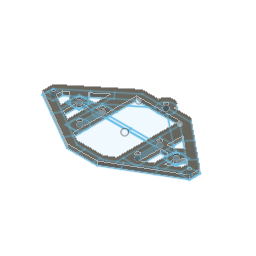
carBodyServoPlate v2 (Autodesk Fusion 360 design; units mm, degrees)
Autodesk Fusion 360 part; units mm, degrees
sketch "Sketch1" plane through (0, 0, 0) normal (0, 0, 1) x (1, 0, 0)
  line L0 (-0.0001, 25.5) -> (-0.0001, 31.5)
  circle A0 centre (-0.0001, 31.5) radius 1.65
  circle A1 centre (-0.0001, 31.5) radius 6
  line L1 (37.0364, 2.2639) -> (-37.0366, 2.2639)
  circle A2 centre (37.0364, 2.2639) radius 1.65
  circle A3 centre (-37.0366, 2.2639) radius 1.65
  line L2 (-0.0001, 31.5) -> (37.0364, 2.2639)
  line L3 (-0.0001, 31.5) -> (-37.0366, 2.2639)
  line L4 (56, 1.4) -> (56, -6.6)
  line L5 (-56, -6.6) -> (-56, 1.4)
  line L6 (-18.5, 31.9382) -> (18.5, 31.9382)
  line L7 (11.4999, -32.5) -> (-11.5001, -32.5)
  line L8 (-11.5001, -32.5) -> (-56, -6.6)
  line L9 (11.4999, -32.5) -> (56, -6.6)
  line L10 (56, -2.6) -> (52, -2.6)
  circle A4 centre (52, -2.6) radius 1.1
  line L11 (-56, -2.6) -> (-52, -2.6)
  circle A5 centre (-52, -2.6) radius 1.1
  line L12 (-22.0001, 4.7639) -> (-22.0001, 2.2639)
  line L13 (-0.0001, 2.2639) -> (-22.0001, 2.2639)
  line L14 (-22.0001, 2.2639) -> (-22.0001, 4.7639)
  line L15 (-22.0001, 4.7639) -> (-0.0001, 4.7639)
  line L16 (-0.0001, 4.7639) -> (-0.0001, 2.2639)
  line L17 (-0.0001, 4.7639) -> (21.9999, 4.7639)
  line L18 (21.9999, 4.7639) -> (21.9999, 2.2639)
  line L19 (21.9999, 2.2639) -> (-0.0001, 2.2639)
  line L20 (-0.0001, 2.2639) -> (-0.0001, 4.7639)
  circle A6 centre (-22.0001, 4.7639) radius 1.65
  circle A7 centre (21.9999, 4.7639) radius 1.65
  line L21 (21.9999, 4.7639) -> (21.9999, -12.2361)
  line L22 (-22.0001, 4.7639) -> (-22.0001, -12.2361)
  circle A8 centre (21.9999, -12.2361) radius 1.65
  circle A9 centre (-22.0001, -12.2361) radius 1.65
  circle A10 centre (-22.0001, -12.2361) radius 5.5
  circle A11 centre (-22.0001, 4.7639) radius 5.5
  line L23 (-27.5001, -17.7361) -> (-16.5001, -17.7361)
  line L24 (-16.5001, -17.7361) -> (-16.5001, 10.2639)
  line L25 (-16.5001, 10.2639) -> (-27.5001, 10.2639)
  line L26 (-27.5001, 10.2639) -> (-27.5001, -17.7361)
  line L27 (27.4999, -17.7361) -> (27.4999, 10.2639)
  line L28 (27.4999, 10.2639) -> (16.4999, 10.2639)
  line L29 (16.4999, 10.2639) -> (16.4999, -17.7361)
  line L30 (16.4999, -17.7361) -> (27.4999, -17.7361)
  line L31 (56, -6.6) -> (48, -6.6)
  line L32 (48, -6.6) -> (48, 1.4)
  line L33 (48, 1.4) -> (56, 1.4)
  line L34 (56, 1.4) -> (56, -6.6)
  line L35 (-56, -6.6) -> (-48, -6.6)
  line L36 (-48, -6.6) -> (-48, 1.4)
  line L37 (-48, 1.4) -> (-56, 1.4)
  line L38 (-56, 1.4) -> (-56, -6.6)
  line L39 (-20.5229, -27.2485) -> (-17.5048, -22.0629)
  line L40 (-40.4384, -15.6572) -> (-37.4202, -10.4716)
  line L41 (-17.5048, -22.0629) -> (-37.4202, -10.4716)
  line L42 (-37.4202, -10.4716) -> (-48, -4.3139)
  line L43 (-17.5048, -22.0629) -> (-11.5001, -25.5578)
  line L44 (22.8887, -25.8715) -> (19.8706, -20.6859)
  line L45 (39.4309, -16.2436) -> (36.4127, -11.058)
  line L46 (36.4127, -11.058) -> (19.8706, -20.6859)
  line L47 (36.4127, -11.058) -> (48, -4.3139)
  line L48 (19.8706, -20.6859) -> (11.4999, -25.5578)
  line L49 (56, 1.4) -> (18.5, 31.9382)
  line L50 (45.76, 9.7389) -> (41.9713, 5.0865)
  line L51 (31.8969, 21.0284) -> (28.1081, 16.376)
  line L52 (41.9713, 5.0865) -> (28.1081, 16.376)
  line L53 (28.1081, 16.376) -> (15.6762, 26.5)
  line L54 (41.9713, 5.0865) -> (48, 0.177)
  circle A12 centre (37.0364, 2.2639) radius 5
  line L55 (32.0364, -2.7361) -> (42.0364, -2.7361)
  line L56 (42.0364, -2.7361) -> (42.0364, 7.2639)
  line L57 (42.0364, 7.2639) -> (32.0364, 7.2639)
  line L58 (32.0364, 7.2639) -> (32.0364, -2.7361)
  line L59 (42.0364, -2.7361) -> (37.0364, 2.2639)
  line L60 (32.0364, 7.2639) -> (37.0364, 2.2639)
  line L61 (40.572, -1.2717) -> (44.2431, 3.2364)
  line L62 (33.5009, 5.7994) -> (36.9098, 9.2083)
  line L63 (-56, 1.4) -> (-18.5, 31.9382)
  line L64 (-30.0227, 22.5547) -> (-26.234, 17.9022)
  line L65 (-40.3156, 14.1727) -> (-36.5979, 9.4632)
  line L66 (-26.234, 17.9022) -> (-36.5979, 9.4632)
  line L67 (-36.5979, 9.4632) -> (-48, 0.4625)
  line L68 (-26.234, 17.9022) -> (-15.6762, 26.5)
  line L69 (7.8699, -32.5) -> (7.8699, -26.5)
  line L70 (-4.112, -32.5) -> (-4.112, -26.5)
  line L71 (7.8699, -26.5) -> (-4.112, -26.5)
  line L72 (11.4999, -25.5578) -> (9.881, -26.5)
  line L73 (9.881, -26.5) -> (7.8699, -26.5)
  line L74 (-4.112, -26.5) -> (-9.8811, -26.5)
  line L75 (-9.8811, -26.5) -> (-11.5001, -25.5578)
  line L76 (16.4999, -17.7361) -> (16.4999, -22.6477)
  line L77 (-16.5001, -17.7361) -> (-16.5001, -22.6477)
  line L78 (27.4999, 10.2639) -> (27.4999, 16.8713)
  line L79 (-27.5001, 10.2639) -> (-27.5001, 16.8713)
  line L80 (-0.0001, 25.5) -> (16.9042, 25.5)
  line L81 (16.4999, 10.2639) -> (16.4999, 25.5)
  line L82 (-0.0001, 25.5) -> (-16.9042, 25.5)
  line L83 (-16.5001, 10.2639) -> (-16.5001, 25.5)
  line L84 (-42.0366, 7.2639) -> (-37.0366, 7.2639)
  line L85 (-37.0366, 7.2639) -> (-37.0366, 2.2639)
  line L86 (-32.0366, -2.7361) -> (-42.0366, -2.7361)
  line L87 (-42.0366, -2.7361) -> (-42.0366, 7.2639)
  line L88 (-42.0366, 7.2639) -> (-32.0366, 7.2639)
  line L89 (-32.0366, 7.2639) -> (-32.0366, -2.7361)
  line L90 (-32.0366, 7.2639) -> (-42.0366, -2.7361)
  circle A13 centre (-37.0366, 2.2639) radius 5
  line L91 (-33.501, 5.7994) -> (-36.9147, 9.2131)
  line L92 (-40.5721, -1.2717) -> (-44.8181, 2.9743)
  line L93 (37.0364, -2.7361) -> (34.5364, -2.7361)
  line L94 (37.0364, -2.7361) -> (39.5364, -2.7361)
  line L95 (39.5364, -2.7361) -> (39.5364, -9.2399)
  line L96 (39.5364, -2.7361) -> (39.5364, -2.0663)
  line L97 (34.5364, -2.7361) -> (34.5364, -2.0663)
  line L98 (34.5364, -2.7361) -> (34.5364, -12.15)
  line L99 (32.0364, 2.2639) -> (32.0364, 4.7639)
  line L100 (32.0364, 4.7639) -> (27.4999, 4.7639)
  line L101 (32.0364, 2.2639) -> (32.0364, -0.2361)
  line L102 (32.0364, -0.2361) -> (27.4999, -0.2361)
  line L103 (32.0364, -0.2361) -> (32.7063, -0.2361)
  line L104 (32.0364, 4.7639) -> (32.7063, 4.7639)
  line L105 (-32.0366, -0.2361) -> (-27.5001, -0.2361)
  line L106 (-32.0366, 4.7639) -> (-27.5001, 4.7639)
  line L107 (-32.0366, 4.7639) -> (-32.7064, 4.7639)
  line L108 (-32.0366, -0.2361) -> (-32.7064, -0.2361)
  line L109 (-37.0366, -2.7361) -> (-39.5366, -2.7361)
  line L110 (-37.0366, -2.7361) -> (-34.5366, -2.7361)
  line L111 (-34.5366, -2.7361) -> (-34.5366, -12.15)
  line L112 (-39.5366, -2.7361) -> (-39.5366, -9.2398)
  line L113 (23.6499, -12.2361) -> (20.3499, -12.2361)
  line L114 (20.3499, -12.2361) -> (20.3499, 4.7639)
  line L115 (20.3499, 4.7639) -> (23.6499, 4.7639)
  line L116 (23.6499, 4.7639) -> (23.6499, -12.2361)
  line L117 (-20.3501, -12.2361) -> (-23.6501, -12.2361)
  line L118 (-23.6501, -12.2361) -> (-23.6501, 4.7639)
  line L119 (-23.6501, 4.7639) -> (-20.3501, 4.7639)
  line L120 (-20.3501, 4.7639) -> (-20.3501, -12.2361)
  line L121 (-34.5366, -2.7361) -> (-34.5366, -2.0663)
  line L122 (-39.5366, -2.7361) -> (-39.5366, -2.0663)
  dimension "d3" = 6
  dimension "d4" = 3.3
  dimension "d5" = 12
  dimension "d20" = 3.3
  dimension "d21" = 3.3
  dimension "d24" = 112
  dimension "d25" = 8
  dimension "d26" = 37
  dimension "d30" = 2.2
  dimension "d31" = 4
  dimension "d32" = 4
  dimension "d33" = 2.2
  dimension "d36" = 22
  dimension "d37" = 2.5
  dimension "d38" = 22
  dimension "d39" = 2.5
  dimension "d41" = 3.3
  dimension "d42" = 3.3
  dimension "d58" = 17
  dimension "d59" = 17
  dimension "d60" = 3.3
  dimension "d61" = 3.3
  dimension "d62" = 11
  dimension "d63" = 11
  dimension "d64" = 8
  dimension "d65" = 8
  dimension "d66" = 6
  dimension "d67" = 6
  dimension "d68" = 6
  dimension "d69" = 6
  dimension "d70" = 6
  dimension "d71" = 6
  dimension "d72" = 10
  dimension "d73" = 6
  dimension "d74" = 6
  dimension "d75" = 6
  dimension "d76" = 6
  dimension "d79" = 5
  dimension "d82" = 10
  dimension "d83" = 2.5
  dimension "d84" = 2.5
  dimension "d85" = 2.5
  dimension "d86" = 2.5
  dimension "d87" = 2.5
  dimension "d88" = 2.5
  constraint coincident L0.end A0.centre
  constraint coincident L1.start A2.centre
  constraint coincident L1.end A3.centre
  constraint vertical L4
  constraint vertical L5
  constraint horizontal L6
  constraint horizontal L7
  constraint midpoint L4 L10.start
  constraint perpendicular L4 L10
  constraint coincident L10.end A4.centre
  constraint midpoint L5 L11.start
  constraint perpendicular L5 L11
  constraint coincident L11.end A5.centre
  constraint coincident L1 L12.end
  constraint perpendicular L1 L12
  constraint horizontal L13
  constraint vertical L14
  constraint horizontal L15
  constraint vertical L16
  constraint midpoint L1 L13.start
  constraint horizontal L17
  constraint vertical L18
  constraint horizontal L19
  constraint vertical L20
  constraint coincident L17.end L18.start
  constraint perpendicular L1 L21
  constraint coincident L12.start L14.end
  constraint perpendicular L13 L22
  constraint coincident L21.end A8.centre
  constraint coincident L22.end A9.centre
  constraint concentric A9 A10
  constraint concentric A6 A11
  constraint horizontal L23
  constraint vertical L24
  constraint horizontal L25
  constraint vertical L26
  constraint horizontal L30
  constraint vertical L27
  constraint horizontal L28
  constraint vertical L29
  constraint horizontal L31
  constraint vertical L32
  constraint horizontal L33
  constraint vertical L34
  constraint horizontal L35
  constraint vertical L36
  constraint horizontal L37
  constraint vertical L38
  constraint coincident L8 L39.start
  constraint perpendicular L8 L39
  constraint coincident L8 L40.start
  constraint perpendicular L8 L40
  constraint perpendicular L40 L41
  constraint coincident L36 L42.end
  constraint perpendicular L40 L42
  constraint perpendicular L39 L43
  constraint coincident L9 L44.start
  constraint perpendicular L9 L44
  constraint coincident L9 L45.start
  constraint perpendicular L9 L45
  constraint perpendicular L44 L46
  constraint coincident L32 L47.end
  constraint perpendicular L45 L47
  constraint perpendicular L44 L48
  constraint coincident L49 L50.start
  constraint perpendicular L49 L50
  constraint coincident L49 L51.start
  constraint perpendicular L49 L51
  constraint perpendicular L51 L52
  constraint perpendicular L51 L53
  constraint coincident L32 L54.end
  constraint perpendicular L50 L54
  constraint concentric A2 A12
  constraint horizontal L55
  constraint vertical L56
  constraint horizontal L57
  constraint vertical L58
  constraint parallel L59 L60
  constraint coincident L59 L61.start
  constraint coincident A12 L61.start
  constraint coincident L54 L61.end
  constraint perpendicular L54 L61
  constraint coincident L60 L62.start
  constraint coincident A12 L62.start
  constraint coincident L52 L62.end
  constraint tangent A12 L62
  constraint coincident L63 L64.start
  constraint perpendicular L63 L64
  constraint coincident L63 L65.start
  constraint perpendicular L3 L65
  constraint coincident L36 L67.end
  constraint perpendicular L65 L67
  constraint perpendicular L64 L68
  constraint coincident L7 L69.start
  constraint perpendicular L7 L69
  constraint coincident L7 L70.start
  constraint perpendicular L7 L70
  constraint perpendicular L70 L71
  constraint parallel L9 L72
  constraint perpendicular L69 L73
  constraint perpendicular L70 L74
  constraint parallel L43 L75
  constraint coincident L48 L76.end
  constraint perpendicular L30 L76
  constraint coincident L43 L77.end
  constraint perpendicular L23 L77
  constraint coincident L53 L78.end
  constraint perpendicular L28 L78
  constraint coincident L66 L79.end
  constraint perpendicular L25 L79
  constraint coincident L53 L80.end
  constraint tangent A1 L80
  constraint coincident L80 L81.end
  constraint perpendicular L80 L81
  constraint coincident L68 L82.end
  constraint tangent A1 L82
  constraint coincident L82 L83.end
  constraint perpendicular L82 L83
  constraint horizontal L84
  constraint vertical L85
  constraint horizontal L86
  constraint vertical L87
  constraint horizontal L88
  constraint vertical L89
  constraint concentric A3 A13
  constraint coincident A13 L91.start
  constraint coincident L90 L91.start
  constraint coincident L67 L91.end
  constraint tangent A13 L91
  constraint perpendicular L90 L91
  constraint coincident A13 L92.start
  constraint coincident L90 L92.start
  constraint coincident L67 L92.end
  constraint tangent A13 L92
  constraint midpoint L55 L93.start
  constraint parallel L55 L93
  constraint parallel L55 L94
  constraint coincident L47 L95.end
  constraint perpendicular L94 L95
  constraint coincident A12 L96.end
  constraint perpendicular L94 L96
  constraint coincident A12 L97.end
  constraint perpendicular L93 L97
  constraint coincident L46 L98.end
  constraint perpendicular L93 L98
  constraint midpoint L58 L99.start
  constraint perpendicular L1 L99
  constraint coincident L27 L100.end
  constraint perpendicular L27 L100
  constraint perpendicular L100 L101
  constraint coincident L27 L102.end
  constraint perpendicular L27 L102
  constraint coincident A12 L103.end
  constraint perpendicular L58 L103
  constraint coincident A12 L104.end
  constraint perpendicular L99 L104
  constraint coincident L89 L105.start
  constraint coincident L26 L105.end
  constraint perpendicular L26 L105
  constraint coincident L89 L106.start
  constraint coincident L26 L106.end
  constraint coincident A11 L106.end
  constraint perpendicular L26 L106
  constraint coincident A13 L107.end
  constraint perpendicular L89 L107
  constraint coincident A13 L108.end
  constraint perpendicular L89 L108
  constraint midpoint L86 L109.start
  constraint perpendicular L26 L109
  constraint parallel L86 L110
  constraint coincident L41 L111.end
  constraint perpendicular L110 L111
  constraint coincident L42 L112.end
  constraint perpendicular L109 L112
  constraint horizontal L113
  constraint vertical L114
  constraint horizontal L115
  constraint vertical L116
  constraint coincident A7 L114.end
  constraint coincident L17 L114.end
  constraint coincident A8 L113.start
  constraint horizontal L117
  constraint vertical L118
  constraint horizontal L119
  constraint vertical L120
  constraint coincident A6 L118.end
  constraint coincident A9 L117.start
  constraint coincident A13 L121.end
  constraint perpendicular L86 L121
  constraint coincident A13 L122.end
  constraint perpendicular L86 L122
  measures "d3" distance of L0.start L0.end
  measures "d4" diameter of A0
  measures "d5" diameter of A1
  measures "d20" diameter of A2
  measures "d21" diameter of A3
  measures "d24" distance of L5.end L4.start
  measures "d25" distance of L5.end L5.start
  measures "d26" distance of L6.start L6.end
  measures "d30" diameter of A4
  measures "d31" distance of L10.start L10.end
  measures "d32" distance of L11.start L11.end
  measures "d33" diameter of A5
  measures "d36" distance of L12.start L15.end
  measures "d37" distance of L13.start L15.end
  measures "d38" distance of L15.end L17.end
  measures "d39" distance of L15.end L13.start
  measures "d41" diameter of A6
  measures "d42" diameter of A7
  measures "d58" distance of L17.end L21.end
  measures "d59" distance of L12.start L22.end
  measures "d60" diameter of A8
  measures "d61" diameter of A9
  measures "d62" diameter of A10
  measures "d63" diameter of A11
  measures "d64" distance of L4.end L31.end
  measures "d65" distance of L5.start L35.end
  measures "d66" distance of L39.start L39.end
  measures "d67" distance of L40.start L40.end
  measures "d68" distance of L44.start L44.end
  measures "d69" distance of L45.start L45.end
  measures "d70" distance of L50.start L50.end
  measures "d71" distance of L51.start L51.end
  measures "d72" diameter of A12
  measures "d73" distance of L64.start L64.end
  measures "d74" distance of L65.start L65.end
  measures "d75" distance of L69.start L69.end
  measures "d76" distance of L70.start L70.end
  measures "d79" distance of L1.end L84.end
  measures "d82" diameter of A13
  measures "d83" distance of L93.start L93.end
  measures "d84" distance of L93.start L94.end
  measures "d85" distance of L99.start L99.end
  measures "d86" distance of L99.start L101.end
  measures "d87" distance of L109.start L109.end
  measures "d88" distance of L109.start L110.end
sketch "Sketch1 (2)" plane through (0, 0, 0) normal (0, 0, 1) x (1, 0, 0) in component "carBodyServoPlate"
  line L0 (11.4999, -32.5) -> (-11.5001, -32.5)
  line L1 (-32.0366, -0.2361) -> (-27.5001, -0.2361)
  line L2 (-26.234, 17.9022) -> (-15.6762, 26.5)
  line L3 (-37.0366, 7.2639) -> (-37.0366, 2.2639)
  line L4 (-48, 1.4) -> (-56, 1.4)
  line L5 (-22.0001, 2.2639) -> (-22.0001, 4.7639)
  line L6 (-40.3156, 14.1727) -> (-36.5979, 9.4632)
  circle A0 centre (-22.0001, 4.7639) radius 1.65
  line L7 (-0.0001, 25.5) -> (-16.9042, 25.5)
  line L8 (-32.0366, 4.7639) -> (-32.7064, 4.7639)
  line L9 (-56, 1.4) -> (-18.5, 31.9382)
  line L10 (-0.0001, 4.7639) -> (21.9999, 4.7639)
  circle A1 centre (-37.0366, 2.2639) radius 1.65
  line L11 (-32.0366, 4.7639) -> (-27.5001, 4.7639)
  line L12 (-42.0366, 7.2639) -> (-32.0366, 7.2639)
  line L13 (-36.5979, 9.4632) -> (-48, 0.4625)
  line L14 (-32.0366, -0.2361) -> (-32.7064, -0.2361)
  line L15 (27.4999, 10.2639) -> (27.4999, 16.8713)
  line L16 (37.0364, -2.7361) -> (34.5364, -2.7361)
  line L17 (39.4309, -16.2436) -> (36.4127, -11.058)
  line L18 (16.4999, -17.7361) -> (16.4999, -22.6477)
  line L19 (32.0364, 2.2639) -> (32.0364, 4.7639)
  line L20 (-34.5366, -2.7361) -> (-34.5366, -2.0663)
  line L21 (32.0364, 2.2639) -> (32.0364, -0.2361)
  line L22 (28.1081, 16.376) -> (15.6762, 26.5)
  circle A2 centre (-22.0001, -12.2361) radius 5.5
  line L23 (-40.4384, -15.6572) -> (-37.4202, -10.4716)
  line L24 (32.0364, -2.7361) -> (42.0364, -2.7361)
  line L25 (45.76, 9.7389) -> (41.9713, 5.0865)
  line L26 (31.8969, 21.0284) -> (28.1081, 16.376)
  line L27 (-34.5366, -2.7361) -> (-34.5366, -12.15)
  line L28 (42.0364, 7.2639) -> (32.0364, 7.2639)
  line L29 (-27.5001, -17.7361) -> (-16.5001, -17.7361)
  line L30 (-4.112, -26.5) -> (-9.8811, -26.5)
  line L31 (27.4999, 10.2639) -> (16.4999, 10.2639)
  line L32 (-20.5229, -27.2485) -> (-17.5048, -22.0629)
  line L33 (-20.3501, -12.2361) -> (-23.6501, -12.2361)
  line L34 (32.0364, 4.7639) -> (27.4999, 4.7639)
  line L35 (39.5364, -2.7361) -> (39.5364, -9.2399)
  circle A3 centre (-52, -2.6) radius 1.1
  circle A4 centre (-22.0001, -12.2361) radius 1.65
  line L36 (32.0364, -0.2361) -> (32.7063, -0.2361)
  line L37 (32.0364, 7.2639) -> (37.0364, 2.2639)
  line L38 (39.5364, -2.7361) -> (39.5364, -2.0663)
  line L39 (7.8699, -32.5) -> (7.8699, -26.5)
  line L40 (-16.5001, -17.7361) -> (-16.5001, -22.6477)
  line L41 (11.4999, -25.5578) -> (9.881, -26.5)
  line L42 (36.4127, -11.058) -> (48, -4.3139)
  line L43 (36.4127, -11.058) -> (19.8706, -20.6859)
  circle A5 centre (21.9999, 4.7639) radius 1.65
  line L44 (-56, -2.6) -> (-52, -2.6)
  circle A6 centre (52, -2.6) radius 1.1
  line L45 (-4.112, -32.5) -> (-4.112, -26.5)
  line L46 (32.0364, 4.7639) -> (32.7063, 4.7639)
  circle A7 centre (37.0364, 2.2639) radius 1.65
  line L47 (34.5364, -2.7361) -> (34.5364, -12.15)
  line L48 (20.3499, 4.7639) -> (23.6499, 4.7639)
  line L49 (-39.5366, -2.7361) -> (-39.5366, -9.2398)
  line L50 (33.5009, 5.7994) -> (36.9098, 9.2083)
  line L51 (23.6499, -12.2361) -> (20.3499, -12.2361)
  line L52 (41.9713, 5.0865) -> (28.1081, 16.376)
  line L53 (-32.0366, 7.2639) -> (-42.0366, -2.7361)
  line L54 (-37.0366, -2.7361) -> (-39.5366, -2.7361)
  line L55 (41.9713, 5.0865) -> (48, 0.177)
  line L56 (-11.5001, -32.5) -> (-56, -6.6)
  line L57 (22.8887, -25.8715) -> (19.8706, -20.6859)
  line L58 (-20.3501, 4.7639) -> (-20.3501, -12.2361)
  line L59 (-23.6501, -12.2361) -> (-23.6501, 4.7639)
  line L60 (-9.8811, -26.5) -> (-11.5001, -25.5578)
  line L61 (-22.0001, 4.7639) -> (-22.0001, -12.2361)
  line L62 (21.9999, 4.7639) -> (21.9999, -12.2361)
  line L63 (-56, -6.6) -> (-56, 1.4)
  line L64 (20.3499, -12.2361) -> (20.3499, 4.7639)
  line L65 (56, 1.4) -> (56, -6.6)
  line L66 (-40.5721, -1.2717) -> (-44.8181, 2.9743)
  line L67 (42.0364, -2.7361) -> (42.0364, 7.2639)
  line L68 (42.0364, -2.7361) -> (37.0364, 2.2639)
  line L69 (-56, 1.4) -> (-56, -6.6)
  line L70 (-32.0366, -2.7361) -> (-42.0366, -2.7361)
  line L71 (-39.5366, -2.7361) -> (-39.5366, -2.0663)
  line L72 (56, 1.4) -> (56, -6.6)
  line L73 (16.4999, -17.7361) -> (27.4999, -17.7361)
  line L74 (-17.5048, -22.0629) -> (-11.5001, -25.5578)
  circle A8 centre (-37.0366, 2.2639) radius 5
  line L75 (56, 1.4) -> (18.5, 31.9382)
  line L76 (-27.5001, 10.2639) -> (-27.5001, -17.7361)
  line L77 (-56, -6.6) -> (-48, -6.6)
  line L78 (-0.0001, 4.7639) -> (-0.0001, 2.2639)
  line L79 (16.4999, 10.2639) -> (16.4999, 25.5)
  line L80 (27.4999, -17.7361) -> (27.4999, 10.2639)
  line L81 (32.0364, 7.2639) -> (32.0364, -2.7361)
  line L82 (-37.4202, -10.4716) -> (-48, -4.3139)
  line L83 (-37.0366, -2.7361) -> (-34.5366, -2.7361)
  line L84 (21.9999, 4.7639) -> (21.9999, 2.2639)
  line L85 (56, -6.6) -> (48, -6.6)
  line L86 (-16.5001, -17.7361) -> (-16.5001, 10.2639)
  line L87 (48, -6.6) -> (48, 1.4)
  line L88 (-17.5048, -22.0629) -> (-37.4202, -10.4716)
  line L89 (-27.5001, 10.2639) -> (-27.5001, 16.8713)
  line L90 (21.9999, 2.2639) -> (-0.0001, 2.2639)
  line L91 (-22.0001, 4.7639) -> (-22.0001, 2.2639)
  line L92 (-23.6501, 4.7639) -> (-20.3501, 4.7639)
  line L93 (-0.0001, 25.5) -> (16.9042, 25.5)
  line L94 (-16.5001, 10.2639) -> (-16.5001, 25.5)
  line L95 (-18.5, 31.9382) -> (18.5, 31.9382)
  line L96 (19.8706, -20.6859) -> (11.4999, -25.5578)
  line L97 (48, 1.4) -> (56, 1.4)
  line L98 (37.0364, -2.7361) -> (39.5364, -2.7361)
  line L99 (11.4999, -32.5) -> (56, -6.6)
  line L100 (40.572, -1.2717) -> (44.2431, 3.2364)
  circle A9 centre (21.9999, -12.2361) radius 1.65
  line L101 (32.0364, -0.2361) -> (27.4999, -0.2361)
  line L102 (34.5364, -2.7361) -> (34.5364, -2.0663)
  line L103 (9.881, -26.5) -> (7.8699, -26.5)
  line L104 (56, -2.6) -> (52, -2.6)
  line L105 (-0.0001, 2.2639) -> (-0.0001, 4.7639)
  line L106 (-26.234, 17.9022) -> (-36.5979, 9.4632)
  line L107 (-0.0001, 25.5) -> (-0.0001, 31.5)
  circle A10 centre (-0.0001, 31.5) radius 1.65
  line L108 (-33.501, 5.7994) -> (-36.9147, 9.2131)
  line L109 (7.8699, -26.5) -> (-4.112, -26.5)
  line L110 (-30.0227, 22.5547) -> (-26.234, 17.9022)
  line L111 (-32.0366, 7.2639) -> (-32.0366, -2.7361)
  line L112 (-22.0001, 4.7639) -> (-0.0001, 4.7639)
  line L113 (-16.5001, 10.2639) -> (-27.5001, 10.2639)
  line L114 (-42.0366, 7.2639) -> (-37.0366, 7.2639)
  circle A11 centre (-0.0001, 31.5) radius 6
  line L115 (-48, -6.6) -> (-48, 1.4)
  line L116 (37.0364, 2.2639) -> (-37.0366, 2.2639)
  line L117 (-42.0366, -2.7361) -> (-42.0366, 7.2639)
  circle A12 centre (-22.0001, 4.7639) radius 5.5
  line L118 (-0.0001, 31.5) -> (-37.0366, 2.2639)
  line L119 (-0.0001, 31.5) -> (37.0364, 2.2639)
  line L120 (23.6499, 4.7639) -> (23.6499, -12.2361)
  line L121 (-0.0001, 2.2639) -> (-22.0001, 2.2639)
  line L122 (16.4999, 10.2639) -> (16.4999, -17.7361)
  circle A13 centre (37.0364, 2.2639) radius 5
  dimension "d93" = 6
  dimension "d94" = 3.3
  dimension "d95" = 12
  dimension "d96" = 3.3
  dimension "d97" = 3.3
  dimension "d98" = 112
  dimension "d99" = 8
  dimension "d100" = 37
  dimension "d101" = 2.2
  dimension "d102" = 4
  dimension "d103" = 4
  dimension "d104" = 2.2
  dimension "d105" = 22
  dimension "d106" = 2.5
  dimension "d107" = 22
  dimension "d108" = 2.5
  dimension "d109" = 3.3
  dimension "d110" = 3.3
  dimension "d111" = 17
  dimension "d112" = 17
  dimension "d113" = 3.3
  dimension "d114" = 3.3
  dimension "d115" = 11
  dimension "d116" = 11
  dimension "d117" = 8
  dimension "d118" = 8
  dimension "d119" = 6
  dimension "d120" = 6
  dimension "d121" = 6
  dimension "d122" = 6
  dimension "d123" = 6
  dimension "d124" = 6
  dimension "d125" = 10
  dimension "d126" = 6
  dimension "d127" = 6
  dimension "d128" = 6
  dimension "d129" = 6
  dimension "d130" = 5
  dimension "d131" = 10
  dimension "d132" = 2.5
  dimension "d133" = 2.5
  dimension "d134" = 2.5
  dimension "d135" = 2.5
  dimension "d136" = 2.5
  dimension "d137" = 2.5
  constraint coincident L107.end A10.centre
  constraint coincident L37.end A7.centre
  constraint coincident L3.end A1.centre
  constraint vertical L65
  constraint vertical L63
  constraint horizontal L95
  constraint horizontal L0
  constraint midpoint L104.start L65
  constraint perpendicular L65 L104
  constraint coincident A6.centre L104.end
  constraint midpoint L44.start L63
  constraint perpendicular L44 L63
  constraint coincident A3.centre L44.end
  constraint coincident L5.start L116
  constraint perpendicular L91 L116
  constraint horizontal L121
  constraint vertical L5
  constraint horizontal L112
  constraint vertical L78
  constraint midpoint L78.end L116
  constraint horizontal L10
  constraint vertical L84
  constraint horizontal L90
  constraint vertical L105
  constraint coincident L10.end A5.centre
  constraint perpendicular L62 L116
  constraint coincident L5.end A0.centre
  constraint perpendicular L61 L121
  constraint coincident L62.end A9.centre
  constraint coincident A2.centre A4.centre
  constraint concentric A2 A4
  constraint concentric A0 A12
  constraint horizontal L29
  constraint vertical L86
  constraint horizontal L113
  constraint vertical L76
  constraint horizontal L73
  constraint vertical L80
  constraint horizontal L31
  constraint vertical L122
  constraint horizontal L85
  constraint vertical L87
  constraint horizontal L97
  constraint vertical L72
  constraint horizontal L77
  constraint vertical L115
  constraint horizontal L4
  constraint vertical L69
  constraint coincident L32.start L56
  constraint perpendicular L32 L56
  constraint coincident L23.start L56
  constraint perpendicular L23 L56
  constraint perpendicular L23 L88
  constraint coincident L82.end L115
  constraint perpendicular L23 L82
  constraint perpendicular L32 L74
  constraint coincident L57.start L99
  constraint perpendicular L57 L99
  constraint coincident L17.start L99
  constraint perpendicular L17 L99
  constraint perpendicular L43 L57
  constraint coincident L42.end L87
  constraint perpendicular L17 L42
  constraint perpendicular L57 L96
  constraint coincident L25.start L75
  constraint perpendicular L25 L75
  constraint coincident L26.start L75
  constraint perpendicular L26 L75
  constraint perpendicular L26 L52
  constraint perpendicular L22 L26
  constraint coincident L55.end L87
  constraint perpendicular L25 L55
  constraint concentric A7 A13
  constraint horizontal L24
  constraint vertical L67
  constraint horizontal L28
  constraint vertical L81
  constraint parallel L37 L68
  constraint coincident L100.start L68
  constraint coincident L100.start A13
  constraint coincident L100.end L55
  constraint perpendicular L55 L100
  constraint coincident L50.start L37
  constraint coincident L50.start A13
  constraint coincident L50.end L52
  constraint tangent L50 A13
  constraint coincident L110.start L9
  constraint perpendicular L9 L110
  constraint coincident L6.start L9
  constraint perpendicular L6 L118
  constraint coincident L13.end L115
  constraint perpendicular L6 L13
  constraint perpendicular L2 L110
  constraint coincident L39.start L0
  constraint perpendicular L0 L39
  constraint coincident L45.start L0
  constraint perpendicular L0 L45
  constraint perpendicular L45 L109
  constraint parallel L41 L99
  constraint perpendicular L39 L103
  constraint perpendicular L30 L45
  constraint parallel L60 L74
  constraint coincident L18.end L96
  constraint perpendicular L18 L73
  constraint coincident L40.end L74
  constraint perpendicular L29 L40
  constraint coincident L15.end L22
  constraint perpendicular L15 L31
  constraint coincident L89.end L106
  constraint perpendicular L89 L113
  constraint coincident L93.end L22
  constraint tangent L93 A11
  constraint coincident L79.end L93
  constraint perpendicular L79 L93
  constraint coincident L7.end L2
  constraint tangent L7 A11
  constraint coincident L94.end L7
  constraint perpendicular L7 L94
  constraint horizontal L114
  constraint vertical L3
  constraint horizontal L70
  constraint vertical L117
  constraint horizontal L12
  constraint vertical L111
  constraint concentric A1 A8
  constraint coincident L108.start A8
  constraint coincident L108.start L53
  constraint coincident L108.end L13
  constraint tangent A8 L108
  constraint perpendicular L53 L108
  constraint coincident L66.start A8
  constraint coincident L66.start L53
  constraint coincident L66.end L13
  constraint tangent L66 A8
  constraint midpoint L16.start L24
  constraint parallel L16 L24
  constraint parallel L24 L98
  constraint coincident L35.end L42
  constraint perpendicular L35 L98
  constraint coincident L38.end A13
  constraint perpendicular L38 L98
  constraint coincident L102.end A13
  constraint perpendicular L16 L102
  constraint coincident L47.end L43
  constraint perpendicular L16 L47
  constraint midpoint L19.start L81
  constraint perpendicular L19 L116
  constraint coincident L34.end L80
  constraint perpendicular L34 L80
  constraint perpendicular L21 L34
  constraint coincident L101.end L80
  constraint perpendicular L80 L101
  constraint coincident L36.end A13
  constraint perpendicular L36 L81
  constraint coincident L46.end A13
  constraint perpendicular L19 L46
  constraint coincident L1.start L111
  constraint coincident L1.end L76
  constraint perpendicular L1 L76
  constraint coincident L8.start L111
  constraint coincident L11.end L76
  constraint coincident L11.end A12
  constraint perpendicular L11 L76
  constraint coincident L8.end A8
  constraint perpendicular L8 L111
  constraint coincident L14.end A8
  constraint perpendicular L14 L111
  constraint midpoint L54.start L70
  constraint perpendicular L54 L76
  constraint parallel L70 L83
  constraint coincident L27.end L88
  constraint perpendicular L27 L83
  constraint coincident L49.end L82
  constraint perpendicular L49 L54
  constraint horizontal L51
  constraint vertical L64
  constraint horizontal L48
  constraint vertical L120
  constraint coincident L48.start A5
  constraint coincident L48.start L10
  constraint coincident L51.start A9
  constraint horizontal L33
  constraint vertical L59
  constraint horizontal L92
  constraint vertical L58
  constraint coincident L59.end A0
  constraint coincident L33.start A4
  constraint coincident L20.end A8
  constraint perpendicular L20 L70
  constraint coincident L71.end A8
  constraint perpendicular L70 L71
  measures "d93" distance of L7.start L107.end
  measures "d94" diameter of A10
  measures "d95" diameter of A11
  measures "d96" diameter of A7
  measures "d97" diameter of A1
  measures "d98" distance of L4.end L65.start
  measures "d99" distance of L4.end L56.end
  measures "d100" distance of L75.end L9.end
  measures "d101" diameter of A6
  measures "d102" distance of L104.start A6.centre
  measures "d103" distance of L44.start A3.centre
  measures "d104" diameter of A3
  measures "d105" distance of L10.start L5.end
  measures "d106" distance of L78.end L10.start
  measures "d107" distance of L10.end L10.start
  measures "d108" distance of L78.end L10.start
  measures "d109" diameter of A0
  measures "d110" diameter of A5
  measures "d111" distance of L10.end L62.end
  measures "d112" distance of L5.end A2.centre
  measures "d113" diameter of A9
  measures "d114" diameter of A4
  measures "d115" diameter of A2
  measures "d116" diameter of A12
  measures "d117" distance of L85.end L65.end
  measures "d118" distance of L77.end L56.end
  measures "d119" distance of L32.start L32.end
  measures "d120" distance of L23.start L23.end
  measures "d121" distance of L57.start L43.end
  measures "d122" distance of L17.start L17.end
  measures "d123" distance of L25.end L25.start
  measures "d124" distance of L22.start L26.start
  measures "d125" diameter of A13
  measures "d126" distance of L110.start L2.start
  measures "d127" distance of L6.start L6.end
  measures "d128" distance of L39.end L39.start
  measures "d129" distance of L45.start L30.start
  measures "d130" distance of L3.start L3.end
  measures "d131" diameter of A8
  measures "d132" distance of L16.start L16.end
  measures "d133" distance of L35.start L16.start
  measures "d134" distance of L19.start L19.end
  measures "d135" distance of L21.end L19.start
  measures "d136" distance of L49.start L54.start
  measures "d137" distance of L54.start L20.start
extrude "Extrude2" add sketch "Sketch1 (2)" along normal blind 3 contours L0 L39 L41 L57 L96 L99 L103 | L0 L39 L45 L109 | L17 L43 L57 L73 L80 L99 | L0 L30 L32 L45 L56 L60 L74 | L18 L43 L73 L96 | L17 L42 L85 L87 L99 | L43 L64 L73 L80 L90 A9 L116 L120 L122 | L43 L73 L80 | L16 L24 L35 L42 L43 L47 L98 | L65 L72 L85 L87 L97 | L23 L29 L32 L56 L76 L88 | L29 L40 L74 L88 | L23 L56 L77 L82 L115 | L21 L80 L81 L101 L116 | L10 L64 L90 L116 L122 | L24 L38 L98 A13 | L16 L24 L102 A13 | L25 L55 L67 L75 L87 L97 | A2 L29 L76 L88 | L29 L76 L88 | L27 L49 L54 L70 L82 L83 L88 | L4 L63 L69 L77 L115 | L10 L31 A5 L80 L116 L119 L120 L122 | L19 L34 L80 L81 L116 | L21 L36 L81 A13 | A7 L68 L116 A13 | L25 L26 L28 L52 L67 L75 | A2 L29 L86 | A2 A4 L58 L59 | A7 L116 L119 A13 | L19 L46 L81 A13 | L86 L116 A12 L121 | A2 L58 L86 L116 A12 L121 | L31 L79 L119 | L67 L100 A13 | L55 L67 L100 | L37 A7 L68 L100 A13 | L25 L55 L67 | L25 L28 L52 L67 | L22 L26 L75 L93 L95 A11 L119 | A2 L59 L76 L116 A12 | L54 L70 L71 A8 | L20 L70 A8 L83 | L4 L6 L9 L12 L13 L114 L115 L117 | L86 L113 A12 | L58 L112 L116 A12 L121 | A0 L59 L112 L116 A12 | L58 L116 A12 L121 | L15 L22 L31 L79 L93 L119 | L28 L52 L55 L67 A13 | L1 L76 L111 L116 | A1 L53 A8 L116 | L6 L9 L106 L110 | L37 A7 L119 A13 | L94 L113 L118 | L76 L113 A12 L118 | L93 A11 L119 | L28 L50 L52 | L28 L50 A13 | L95 A10 A11 L119 | L95 A10 A11 | L59 L116 A12 | L14 A8 L111 | L11 L76 L111 L116 | L76 L116 A12 | L3 A1 L53 A8 | L66 A8 L117 | L13 L66 L117 | L2 L7 L9 L95 L110 A11 L118 | L2 L7 L89 L94 L106 L113 L118 | L7 L94 L118 | L76 L113 L118 | L107 A10 A11 L118 | L7 A11 L118 | L107 A10 A11 L119 | L95 A10 A11 L118 | A1 A8 L116 L118 | L8 A8 L111 | L12 L13 A8 L114 L117 | L12 L13 L114 L117 | L12 L13 L108 L114 | L3 A1 L53 A8 | L12 A8 L108 | A1 L53 A8 L118 in component "carBodyServoPlate"
extrude "Extrude3" cut sketch "Sketch1 (2)" along normal blind 3 contours L7 L94 L118 in component "carBodyServoPlate"
extrude "Extrude5" add sketch "Sketch1 (2)" along normal blind 3 contours L31 L80 L119 in component "carBodyServoPlate"
extrude "Extrude6" add sketch "Sketch1 (2)" along normal blind 3 contours L62 L64 L90 A9 L116 | L62 A9 L116 L120 | A2 A4 L58 L61 | A2 L58 L61 A12 | A2 L59 L61 A12 | A2 A4 L59 L61 | L58 L61 L116 A12 L121 | L59 L61 L116 A12 in component "carBodyServoPlate"
extrude "Extrude7" add sketch "Sketch1 (2)" along normal blind 3 contours A5 L62 L64 L84 L90 L116 | A5 L62 L84 L116 L120 in component "carBodyServoPlate"
component "carBodyServoPlate" placed x (1, 0, 0) y (0, 1, 0) z (0, 0, 1) at (0, 0, 0)
